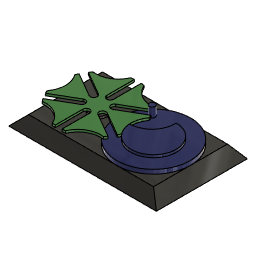
Geneva Drive Mechanism (Autodesk Fusion 360 design; units mm, degrees)
Autodesk Fusion 360 part; units mm, degrees
sketch "Bottom of base" plane through (0, 0, 0) normal (0, 0, 1) x (1, 0, 0) in component "Base"
  line L0 (75, -40) -> (-55, -40)
  line L1 (-55, 40) -> (75, 40)
  line L2 (75, 40) -> (75, -40)
  line L3 (75, -40) -> (0, 0) construction
  line L4 (0, 0) -> (75, 40) construction
  line L5 (75, -40) -> (-55, -40)
  line L6 (-55, 40) -> (75, 40)
  line L7 (75, 40) -> (75, -40)
  line L8 (75, -40) -> (-55, -40)
  line L9 (-55, -40) -> (-55, 40)
  line L10 (-55, 40) -> (75, 40)
  line L11 (75, 40) -> (75, -40)
  line L12 (0, 0) -> (-55, 40) construction
  line L13 (0, 0) -> (-55, -40) construction
  dimension "d103" = 130
  constraint horizontal L0
  constraint parallel L0 L1
  constraint coincident L3 L4.start
  constraint coincident L4 L3.end
  constraint coincident L3.end L4.start
  constraint horizontal L5
  constraint horizontal L6
  constraint vertical L7
  constraint horizontal L8
  constraint vertical L9
  constraint horizontal L10
  constraint vertical L11
  measures "d103" distance of L0.start L0.end
ref_plane "WorkPlane1" through (10, 0, 10) normal (0, 0, 1) x (1, 0, 0) in component "Base"
sketch "Top of base" plane through (0, 0, 10) normal (0, 0, 1) x (1, 0, 0) in component "Base"
  line L0 (65, -32.5) -> (-45, -32.5)
  line L1 (-45, 32.5) -> (65, 32.5)
  line L2 (65, 32.5) -> (65, -32.5)
  line L3 (65, -32.5) -> (0, 0) construction
  line L4 (0, 0) -> (65, 32.5) construction
  line L5 (65, -32.5) -> (-45, -32.5)
  line L6 (-45, 32.5) -> (65, 32.5)
  line L7 (65, 32.5) -> (65, -32.5)
  line L8 (65, -32.5) -> (-45, -32.5)
  line L9 (-45, -32.5) -> (-45, 32.5)
  line L10 (-45, 32.5) -> (65, 32.5)
  line L11 (65, 32.5) -> (65, -32.5)
  line L12 (0, 0) -> (-45, 32.5) construction
  line L13 (0, 0) -> (-45, -32.5) construction
  dimension "d104" = 110
  constraint horizontal L0
  constraint parallel L0 L1
  constraint coincident L3 L4.start
  constraint coincident L4 L3.end
  constraint coincident L3.end L4.start
  constraint horizontal L5
  constraint horizontal L6
  constraint vertical L7
  constraint horizontal L8
  constraint vertical L9
  constraint horizontal L10
  constraint vertical L11
  measures "d104" distance of L0.start L0.end
loft "Loft1" add profiles "Bottom of base", "Top of base" section 1 section 2 makes body 1 in component "Base"
sketch "Connecting pins" plane through (0, 0, 10) normal (0, 0, 1) x (-1, 0, 0) in component "Base"
  circle A0 centre (-32.5, 0) radius 5
  circle A1 centre (16.25, 0) radius 5
  circle A2 centre (16.25, 0) radius 7.5
  line L0 (-65, -32.5) -> (45, -32.5)
  line L1 (45, -32.5) -> (45, 32.5)
  line L2 (45, 32.5) -> (-65, 32.5)
  line L3 (-65, 32.5) -> (-65, -32.5)
  dimension "d6" = 10
  dimension "d7" = 16.25
  dimension "d8" = 10
  dimension "d9" = 15
  constraint concentric A1 A2
  measures "d6" diameter of A0
  measures "d7" distance of origin A1.centre
  measures "d8" diameter of A1
  measures "d9" diameter of A2
extrude "Extrude1" add sketch "Connecting pins" along normal blind 2 contours A2 bodies 1 in component "Base"
extrude "Extrude2" add 1 faces at (-13.5602, -0.0371, 10) along direction (0, 0, 1) blind 5 on bodies 1 bodies 1 in component "Base"
sketch "Flower Crank" plane through (0, 0, 10) normal (0, 0, 1) x (1, 0, 0) in component "Flower Crank"
  line L0 (-16.25, 35) -> (-16.25, -7.5) construction
  circle A0 centre (-16.25, 0) radius 7.5
  line L1 (-13.25, -32) -> (-13.25, -10.5)
  arc A1 (-13.25, -10.5) -> (-19.25, -10.5) centre (-16.25, -10.5) ccw
  line L2 (-19.25, -10.5) -> (-19.25, -32)
  line L3 (-13.25, -29.5353) -> (-13.25, -34.8712)
  line L4 (-19.25, -31.7183) -> (-19.25, -34.8712)
  line L5 (12.9628, -13.4019) -> (-5.6567, -2.6519)
  line L6 (-8.6567, -7.8481) -> (9.9628, -18.5981)
  arc A2 (-5.6567, -2.6519) -> (-8.6567, -7.8481) centre (-7.1567, -5.25) ccw
  line L7 (9.7189, -18.4572) -> (12.4493, -20.0337)
  line L8 (10.8283, -12.1696) -> (15.4493, -14.8375)
  line L9 (9.9628, 18.5981) -> (-8.6567, 7.8481)
  line L10 (-5.6567, 2.6519) -> (12.9628, 13.4019)
  arc A3 (-8.6567, 7.8481) -> (-5.6567, 2.6519) centre (-7.1567, 5.25) ccw
  line L11 (12.7189, 13.2611) -> (15.4493, 14.8375)
  line L12 (7.8283, 17.3657) -> (12.4493, 20.0337)
  line L13 (-19.25, 32) -> (-19.25, 10.5)
  line L14 (-13.25, 10.5) -> (-13.25, 32)
  arc A4 (-19.25, 10.5) -> (-13.25, 10.5) centre (-16.25, 10.5) ccw
  line L15 (-13.25, 31.7183) -> (-13.25, 34.8712)
  line L16 (-19.25, 29.5353) -> (-19.25, 34.8712)
  line L17 (-45.4628, 13.4019) -> (-26.8433, 2.6519)
  line L18 (-23.8433, 7.8481) -> (-42.4628, 18.5981)
  arc A5 (-26.8433, 2.6519) -> (-23.8433, 7.8481) centre (-25.3433, 5.25) ccw
  line L19 (-42.2189, 18.4572) -> (-44.9493, 20.0337)
  line L20 (-43.3283, 12.1696) -> (-47.9493, 14.8375)
  line L21 (-42.4628, -18.5981) -> (-23.8433, -7.8481)
  line L22 (-26.8433, -2.6519) -> (-45.4628, -13.4019)
  arc A6 (-23.8433, -7.8481) -> (-26.8433, -2.6519) centre (-25.3433, -5.25) ccw
  line L23 (-45.2189, -13.2611) -> (-47.9493, -14.8375)
  line L24 (-40.3283, -17.3657) -> (-44.9493, -20.0337)
  arc A7 (16.5865, 12.1145) -> (16.5865, -12.1145) centre (32.5, 0) ccw
  arc A8 (-10.3232, 34.4945) -> (10.6598, 22.38) centre (8.125, 42.2187) ccw
  arc A9 (-43.1598, 22.38) -> (-22.1768, 34.4945) centre (-40.625, 42.2187) ccw
  arc A10 (-49.0865, -12.1145) -> (-49.0865, 12.1145) centre (-65, 0) ccw
  arc A11 (-22.1768, -34.4945) -> (-43.1598, -22.38) centre (-40.625, -42.2187) ccw
  arc A12 (10.6598, -22.38) -> (-10.3232, -34.4945) centre (8.125, -42.2187) ccw
  circle A13 centre (-16.25, 0) radius 5
  arc A14 (16.5865, 12.1145) -> (15.4493, 14.8375) centre (-16.25, 0) ccw
  arc A15 (12.4493, 20.0337) -> (10.6598, 22.38) centre (-16.25, 0) ccw
  arc A16 (10.6598, -22.38) -> (12.4493, -20.0337) centre (-16.25, 0) ccw
  arc A17 (15.4493, -14.8375) -> (16.5865, -12.1145) centre (-16.25, 0) ccw
  arc A18 (-22.1768, -34.4945) -> (-19.25, -34.8712) centre (-16.25, 0) ccw
  arc A19 (-13.25, -34.8712) -> (-10.3232, -34.4945) centre (-16.25, 0) ccw
  arc A20 (-49.0865, -12.1145) -> (-47.9493, -14.8375) centre (-16.25, 0) ccw
  arc A21 (-44.9493, -20.0337) -> (-43.1598, -22.38) centre (-16.25, 0) ccw
  arc A22 (-43.1598, 22.38) -> (-44.9493, 20.0337) centre (-16.25, 0) ccw
  arc A23 (-47.9493, 14.8375) -> (-49.0865, 12.1145) centre (-16.25, 0) ccw
  arc A24 (-10.3232, 34.4945) -> (-13.25, 34.8712) centre (-16.25, 0) ccw
  arc A25 (-19.25, 34.8712) -> (-22.1768, 34.4945) centre (-16.25, 0) ccw
  dimension "d14" = 70
  dimension "d17" = 15
  dimension "d32" = 6
  dimension "d34" = 360
  dimension "d37" = 40
  dimension "d39" = 360
  dimension "d57" = 10
  constraint coincident L0.start A16
  constraint vertical L0
  constraint tangent L1 A1
  constraint tangent A1 L2
  constraint parallel L1 L2
  constraint coincident L1 L3.start
  constraint coincident L3.end A16
  constraint coincident L2 L4.start
  constraint coincident L4.end A16
  constraint coincident A0 L0.end
  constraint coincident A7.start A16
  constraint coincident A8.end A16
  constraint coincident A8.start A16
  constraint coincident A9.end A16
  constraint coincident A9.start A16
  constraint coincident A10.end A16
  constraint coincident A10.start A16
  constraint coincident A11.end A16
  constraint coincident A11.start A16
  constraint concentric A14 A16
  constraint concentric A14 A24
  constraint concentric A22 A24
  constraint concentric A20 A22
  constraint concentric A18 A20
  constraint concentric A13 A24
  constraint concentric A14 A15
  constraint concentric A16 A17
  constraint concentric A18 A19
  constraint concentric A20 A21
  constraint concentric A22 A23
  constraint concentric A24 A25
  measures "d14" diameter of A16
  measures "d17" diameter of A0
  measures "d32" diameter of A1
  measures "d37" diameter of A7
  measures "d57" diameter of A13
sketch "Base Connecting pin" plane through (0, 0, 10) normal (0, 0, 1) x (-1, 0, 0) in component "Circular Crank"
  arc A0 (-18.75, 0.0016) -> (-18.75, 0.0033) centre (-53.75, 0.0033) ccw
  arc A1 (-16.5865, 12.1145) -> (-16.5873, 12.1156) centre (-32.5, 0) ccw
  arc A2 (-18.75, 0.0084) -> (-18.75, 0.0033) centre (16.25, 0.0033) ccw
  line L0 (-18.75, 0.0033) -> (-18.75, 0) construction
  arc A3 (-15.0291, 1.0084) -> (-32.4094, -17.4998) centre (-12.4534, -18.825) ccw
  arc A4 (-13.7868, -17.9664) -> (-13.784, -17.9678) centre (-5, 0) ccw
  arc A5 (-13.7868, 17.9664) -> (-13.7895, 17.9651) centre (-5, 0) ccw
  line L1 (-32.5, 0) -> (-18.75, 0) construction
  line L2 (-32.5, 0) -> (-13.9426, -17.4265) construction
  line L3 (-32.5, 0) -> (-7.043, 0) construction
  arc A6 (-12.5345, 1.1748) -> (-32.4188, -19.9998) centre (-12.4534, -18.825) ccw
  arc A7 (-12.5345, 1.1748) -> (-32.4188, -19.9998) centre (-32.5, 0) ccw
  dimension "d36" = 70
  dimension "d97" = 43.2
  dimension "d99" = 40
  dimension "d100" = 40
  constraint concentric A4 A5
  constraint concentric A1 A7
  constraint tangent A3 A6
  measures "d36" diameter of A2
  measures "d97" angle of L2 L3
  measures "d99" diameter of A7
  measures "d100" diameter of A6
extrude "Extrude1'" add sketch "Flower Crank" along normal blind 6 and the other way blind -4 separate body contours A0 | A0 L5 A2 L8 L10 A3 L11 A7 A14 A17 | A0 L9 A3 L12 L14 A4 L15 A8 A15 A24 | A0 L1 A1 L3 L6 A2 L7 A12 A16 A19 | A0 L13 A4 L16 L18 A5 L19 A9 A22 A25 | A0 A1 L2 L4 L21 A6 L24 A11 A18 A21 | A0 L17 A5 L20 L22 A6 L23 A10 A20 A23 | A13 makes body 2 in component "Flower Crank"
move_face "OffsetFaces1" offset -0.3 2 faces at (-21.2252, 0.4978, 14) (-13.5602, -0.0371, 15) on bodies 1 in component "Base"
sketch "Circular Crank" plane through (0, 0, 10) normal (0, 0, 1) x (-1, 0, 0) in component "Circular Crank"
  circle A0 centre (16.25, 0) radius 7.5
  circle A1 centre (-32.5, 0) radius 32.5
  circle A2 centre (-32.5, 0) radius 5
  line L0 (-65, -32.5) -> (45, -32.5)
  line L1 (45, -32.5) -> (45, 32.5)
  line L2 (45, 32.5) -> (-65, 32.5)
  line L3 (-65, 32.5) -> (-65, -32.5)
  dimension "d45" = 65
  dimension "d64" = 10
  constraint concentric A1 A2
  measures "d45" diameter of A1
  measures "d64" diameter of A2
sketch "Flower Connecting Pin" plane through (0, 0, 10) normal (0, 0, 1) x (-1, 0, 0) in component "Circular Crank"
  circle A0 centre (-13.949, -17.4336) radius 2.9
  line L0 (-13.949, -17.4336) -> (-32.5, 0) construction
  dimension "d76" = 5.8
  constraint coincident A0.centre L0.start
  measures "d76" diameter of A0
extrude "Extrude3" cut sketch "Flower Crank" along normal blind 5 contours A13 bodies 2 in component "Flower Crank"
extrude "Extrude3'" add sketch "Connecting pins" along normal blind 5 contours A0 bodies 1 in component "Base"
extrude "Extrude3''" add sketch "Circular Crank" along normal blind 3.7 separate body contours A1 makes body 3 in component "Circular Crank"
move_face "OffsetFaces2" offset -0.3 1 faces at (27.5062, 0.2492, 13.3333) on bodies 1 in component "Base"
extrude "Extrude4" add sketch "Base Connecting pin" along normal blind 6 contours A0 A1 A3 A6 A7 | A0 A1 A3 A6 A7 bodies 3 in component "Circular Crank"
extrude "Extrude5" cut sketch "Circular Crank" along normal blind 5 contours A2 bodies 3 in component "Circular Crank"
extrude "Extrude6" add sketch "Flower Connecting Pin" along normal blind 12 bodies 3 in component "Circular Crank"
move_face "OffsetFaces1'" offset -0.3 1 faces at (11.0635, 17.1448, 16.4667) on bodies 3 in component "Circular Crank"
component "Base" placed x (1, 0, 0) y (0, 1, 0) z (0, 0, 1) at (0, 0, 0)
component "Flower Crank" placed x (1, 0, 0) y (0, 1, 0) z (0, 0, 1) at (0, 0, 0)
component "Circular Crank" placed x (1, 0, 0) y (0, 1, 0) z (0, 0, 1) at (0, 0, 0)
equation "d7 = ( 65 / 4 ) * 1 mm"
named bodies: "Base", "Flower Crank", "Circular Crank"
